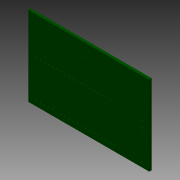
# Autodesk Inventor part: schematic.kicad_pcb
Saved by Autodesk Inventor 2015 SP2 (Build 190223200, 223)
## iProperties
Created: 2016-04-07
Part Number: schematic.kicad_pcb
Material: Generic
Document SubType Name: Modeling
Designer: HP
Density: 1 g/cm^3
Appearance: Board Outline
Author: HP
Autodesk Inventor part; units mm, degrees
ref_plane "YZ Plane" through (0, 0, 0) normal (1, 0, 0) x (0, 1, 0)
ref_plane "XZ Plane" through (0, 0, 0) normal (0, 1, 0) x (-1, 0, 0)
ref_plane "XY Plane" through (0, 0, 0) normal (0, 0, 1) x (1, 0, 0)
sketch "Sketch1" plane through (0, 0, 0) normal (0, 0, 1) x (1, 0, 0)
  line L0 (220.5674, -91.5924) -> (145.5674, -91.5924)
  line L1 (145.5674, -91.5924) -> (145.5674, -140.8874)
  line L2 (145.5674, -140.8874) -> (220.5674, -140.8874)
  line L3 (220.5674, -140.8874) -> (220.5674, -91.5924)
  circle A0 centre (150.4442, -137.3022) radius 0.545
  circle A1 centre (152.9842, -137.3022) radius 0.545
  circle A2 centre (155.5242, -137.3022) radius 0.545
  circle A3 centre (158.0642, -137.3022) radius 0.545
  circle A4 centre (160.6042, -137.3022) radius 0.545
  circle A5 centre (163.1442, -137.3022) radius 0.545
  circle A6 centre (165.6842, -137.3022) radius 0.545
  circle A7 centre (168.2242, -137.3022) radius 0.545
  circle A8 centre (170.7642, -137.3022) radius 0.545
  circle A9 centre (173.3042, -137.3022) radius 0.545
  circle A10 centre (175.8442, -137.3022) radius 0.545
  circle A11 centre (178.3842, -137.3022) radius 0.545
  circle A12 centre (180.9242, -137.3022) radius 0.545
  circle A13 centre (183.4642, -137.3022) radius 0.545
  circle A14 centre (186.0042, -137.3022) radius 0.545
  circle A15 centre (188.5442, -137.3022) radius 0.545
  circle A16 centre (191.0842, -137.3022) radius 0.545
  circle A17 centre (193.6242, -137.3022) radius 0.545
  circle A18 centre (196.1642, -137.3022) radius 0.545
  circle A19 centre (198.7042, -137.3022) radius 0.545
  circle A20 centre (198.7042, -114.4422) radius 0.545
  circle A21 centre (196.1642, -114.4422) radius 0.545
  circle A22 centre (193.6242, -114.4422) radius 0.545
  circle A23 centre (191.0842, -114.4422) radius 0.545
  circle A24 centre (188.5442, -114.4422) radius 0.545
  circle A25 centre (186.0042, -114.4422) radius 0.545
  circle A26 centre (183.4642, -114.4422) radius 0.545
  circle A27 centre (180.9242, -114.4422) radius 0.545
  circle A28 centre (178.3842, -114.4422) radius 0.545
  circle A29 centre (175.8442, -114.4422) radius 0.545
  circle A30 centre (173.3042, -114.4422) radius 0.545
  circle A31 centre (170.7642, -114.4422) radius 0.545
  circle A32 centre (168.2242, -114.4422) radius 0.545
  circle A33 centre (165.6842, -114.4422) radius 0.545
  circle A34 centre (163.1442, -114.4422) radius 0.545
  circle A35 centre (160.6042, -114.4422) radius 0.545
  circle A36 centre (158.0642, -114.4422) radius 0.545
  circle A37 centre (155.5242, -114.4422) radius 0.545
  circle A38 centre (152.9842, -114.4422) radius 0.545
  circle A39 centre (150.4442, -114.4422) radius 0.545
  circle A40 centre (150.6982, -103.251) radius 0.381
  circle A41 centre (153.2382, -103.251) radius 0.381
  circle A42 centre (155.7782, -103.251) radius 0.381
  circle A43 centre (158.3182, -103.251) radius 0.381
  circle A44 centre (150.6982, -95.631) radius 0.381
  circle A45 centre (153.2382, -95.631) radius 0.381
  circle A46 centre (155.7782, -95.631) radius 0.381
  circle A47 centre (158.3182, -95.631) radius 0.381
  circle A48 centre (215.9737, -137.541) radius 0.5
  circle A49 centre (215.9737, -133.911) radius 0.5
  circle A50 centre (215.9737, -130.281) radius 0.5
  circle A51 centre (215.9737, -126.651) radius 0.5
  circle A52 centre (215.9737, -123.021) radius 0.5
  circle A53 centre (215.9737, -119.391) radius 0.5
  circle A54 centre (215.9737, -115.761) radius 0.5
  circle A55 centre (215.9737, -112.131) radius 0.5
  circle A56 centre (215.9737, -108.501) radius 0.5
  circle A57 centre (215.9737, -104.871) radius 0.5
  circle A58 centre (189.1792, -99.695) radius 0.5005
  circle A59 centre (179.0192, -99.695) radius 0.5005
  constraints: 60 centre point, 8 end point
extrude "schematic.kicad_pcb_Outline" add sketch "Sketch1" along normal blind 1.6
body "Solid1"
